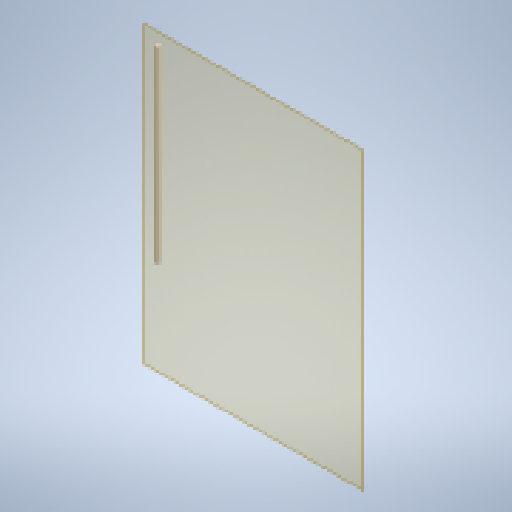
# Autodesk Inventor part: BarraMarco1.2
Saved by Autodesk Inventor 2024 (Build 280153000, 153)
## iProperties
Created: 2023-07-05
Part Number: BarraMarco1.2
Material: Genérico
Document SubType Name: Modeling
Designer: sergi
Density: 1 g/cm^3
Appearance: Valor por defecto
Author: sergi
Autodesk Inventor part; units mm, degrees
ref_plane "YZ Plane" through (0, 0, 0) normal (1, 0, 0) x (0, 1, 0)
ref_plane "XZ Plane" through (0, 0, 0) normal (0, 1, 0) x (-1, 0, 0)
ref_plane "XY Plane" through (0, 0, 0) normal (0, 0, 1) x (1, 0, 0)
ref_plane "Plano de trabajo1" through (0, 0, 0) normal (0, 0, 1) x (1, 0, 0)
sketch "Boceto1" plane through (0, 0, 0) normal (0, 0, 1) x (1, 0, 0)
  line L0 (-706.5, 15) -> (-706.5, 1360) projected
  line L1 (-706.5, 1360) -> (-185.5, 1360) projected
  line L2 (-185.5, 1360) -> (-185.5, 15) projected
  line L3 (-185.5, 15) -> (-706.5, 15) projected
  line L4 (692.5, -15) -> (692.5, -536) projected
  line L5 (692.5, -536) -> (-706.5, -536) projected
  line L6 (-706.5, -536) -> (-706.5, -15) projected
  line L7 (-706.5, -15) -> (692.5, -15) projected
  line L8 (722.5, -566) -> (722.5, 15) projected
  line L9 (722.5, 15) -> (-155.5, 15) projected
  line L10 (-155.5, 15) -> (-155.5, 1390) projected
  line L11 (-155.5, 1390) -> (-736.5, 1390) projected
  line L12 (-736.5, 1390) -> (-736.5, -566) projected
  line L13 (-736.5, -566) -> (722.5, -566) projected
  line L14 (-706.5, 15) -> (-706.5, 45)
  line L15 (-706.5, 45) -> (-185.5, 45)
  line L16 (-185.5, 15) -> (-155.5, 15)
  line L17 (-706.5, 15) -> (-736.5, 15)
  line L18 (-706.5, 1360) -> (-706.5, 1390)
  point P0 (0, 0)
  dimension "d0" = 30
  constraints: 10 end point, 5 point on line, 2 perpendicular, 1 horizontal
  measures "d0" distance of L0.start L14.end
extrude "Extrusión1" add sketch "Boceto1" against normal blind 30 contours L17 L12 L11 L18 L0
